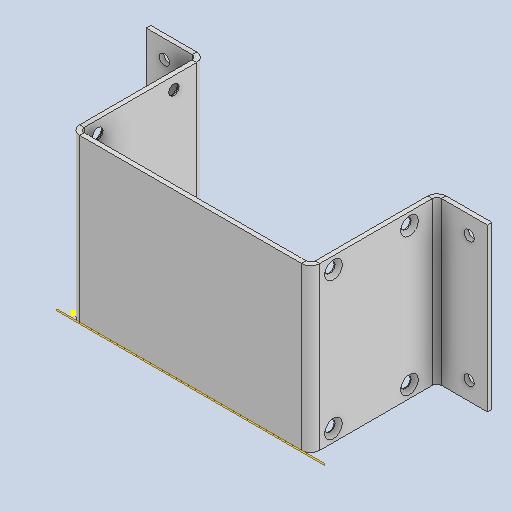
# Autodesk Inventor part: Top
Saved by Autodesk Inventor 2024 (Build 280153000, 153)
## iProperties
Created: 2025-10-29
Part Number: Top
Material: 일반
Document SubType Name: Sheet Metal
Designer: alexi
Density: 1 g/cm^3
Appearance: 기본값
Sheet Metal Rule: 기본값
Author: alexi
Autodesk Inventor part; units mm, degrees
ref_plane "YZ Plane" through (0, 0, 0) normal (1, 0, 0) x (0, 1, 0)
ref_plane "XZ Plane" through (0, 0, 0) normal (0, 1, 0) x (-1, 0, 0)
ref_plane "XY Plane" through (0, 0, 0) normal (0, 0, 1) x (1, 0, 0)
ref_plane "작업 평면1" through (0, 0, 0) normal (0, 0, 1) x (1, 0, 0)
sketch "스케치1" plane through (0, 0, 0) normal (0, 0, 1) x (1, 0, 0)
  line L0 (80, 11.5982) -> (80.0982, 11.5982) projected
  line L1 (80.0982, 41.5982) -> (80, 41.5982) projected
  line L2 (0, 41.5982) -> (-0.0982, 41.5982) projected
  line L3 (5, -0.0088) -> (3.5, -0.0088)
  line L4 (3.5, -0.0088) -> (3.5, 53.2053)
  line L5 (3.5, 53.2053) -> (5, 53.2053)
  line L6 (5, 53.2053) -> (5, -0.0088)
  line L7 (3.5, -0.0088) -> (0, -0.0088)
  line L8 (0, -0.0088) -> (0, 53.2053)
  line L9 (0, 53.2053) -> (3.5, 53.2053)
  line L10 (3.5, 53.2053) -> (3.5, -0.0088)
  line L11 (0, -0.0088) -> (-36.9, -0.0088)
  line L12 (-36.9, -0.0088) -> (-36.9, 53.2053)
  line L13 (-36.9, 53.2053) -> (0, 53.2053)
  line L14 (0, 53.2053) -> (0, -0.0088)
  line L15 (5, 53.2053) -> (5, -0.0088)
  line L16 (75, -0.0088) -> (76.5, -0.0088)
  line L17 (76.5, -0.0088) -> (76.5, 53.2053)
  line L18 (76.5, 53.2053) -> (75, 53.2053)
  line L19 (75, 53.2053) -> (75, -0.0088)
  line L20 (76.5, -0.0088) -> (80, -0.0088)
  line L21 (80, -0.0088) -> (80, 53.2053)
  line L22 (80, 53.2053) -> (76.5, 53.2053)
  line L23 (76.5, 53.2053) -> (76.5, -0.0088)
  line L24 (80, -0.0088) -> (116.9, -0.0088)
  line L25 (116.9, -0.0088) -> (116.9, 53.2053)
  line L26 (116.9, 53.2053) -> (80, 53.2053)
  line L27 (80, 53.2053) -> (80, -0.0088)
  line L28 (5, -0.0088) -> (75, -0.0088) projected
  line L29 (75, 53.2053) -> (5, 53.2053) projected
  line L30 (-36.9, -0.0088) -> (-40.4, -0.0088)
  line L31 (-40.4, -0.0088) -> (-40.4, 53.2053)
  line L32 (-40.4, 53.2053) -> (-36.9, 53.2053)
  line L33 (-36.9, 53.2053) -> (-36.9, -0.0088)
  line L34 (-40.4, -0.0088) -> (-55.4, -0.0088)
  line L35 (-55.4, -0.0088) -> (-55.4, 53.2053)
  line L36 (-55.4, 53.2053) -> (-40.4, 53.2053)
  line L37 (-40.4, 53.2053) -> (-40.4, -0.0088)
  line L38 (116.9, -0.0088) -> (120.4, -0.0088)
  line L39 (120.4, -0.0088) -> (120.4, 53.2053)
  line L40 (120.4, 53.2053) -> (116.9, 53.2053)
  line L41 (116.9, 53.2053) -> (116.9, -0.0088)
  line L42 (120.4, -0.0088) -> (135.4, -0.0088)
  line L43 (135.4, -0.0088) -> (135.4, 53.2053)
  line L44 (135.4, 53.2053) -> (120.4, 53.2053)
  line L45 (120.4, 53.2053) -> (120.4, -0.0088)
  point P0 (0, 0)
  dimension "d0" = 1.5
  dimension "d1" = 3.5
  dimension "d2" = 36.9
  dimension "d3" = 1.5
  dimension "d4" = 3.5
  dimension "d5" = 36.9
  dimension "d33" = 3.5
  dimension "d34" = 3.5
  dimension "d35" = 15
  dimension "d36" = 15
  constraints: 82 end point, 21 equal length, 10 horizontal, 10 perpendicular, 6 point on line
  measures "d0" distance of L5.end L4.end
  measures "d1" distance of L8.end L9.end
  measures "d2" distance of L12.end L13.end
  measures "d3" distance of L18.end L17.end
  measures "d4" distance of L21.end L22.end
  measures "d5" distance of L21.end L25.end
  measures "d33" distance of L12.end L31.end
  measures "d34" distance of L39.end L40.end
  measures "d35" distance of L35.end L36.end
  measures "d36" distance of L43.end L44.end
extrude "판1" add sketch "스케치1" against normal blind 1.5
sketch "스케치2" plane through (0, 0, -1.5) normal (0, 0, -1) x (-1, 0, 0)
  line L0 (-5, 53.2053) -> (-5, -0.0088) projected
  line L1 (-3.5, -0.0088) -> (-3.5, 53.2053) projected
  line L2 (-75, 53.2053) -> (-75, -0.0088) projected
  line L3 (-76.5, 53.2053) -> (-76.5, -0.0088) projected
  point P0 (0, 0)
  constraints: 1 other
fold "접기3" angle 90 bend radius 1.5 thickness 1.5 k factor 0.44 line from (-36.9, -0.0088, 0) to (-36.9, 53.2053, 0) line at bend start moving side (-1, 0, 0) folds toward (0, 0, 1)
fold "접기4" angle 90 bend radius 1.5 thickness 1.5 k factor 0.44 line from (116.9, -0.0088, 0) to (116.9, 53.2053, 0) line at bend start moving side (1, 0, 0) folds toward (0, 0, 1)
fold "접기5" angle 90 bend radius 1.5 thickness 1.5 k factor 0.44 line from (76.5, 53.2053, -1.5) to (76.5, -0.0088, -1.5) line at bend start moving side (1, 0, 0) folds toward (0, 0, -1)
fold "접기6" angle 90 bend radius 1.5 thickness 1.5 k factor 0.44 line from (3.5, -0.0088, -1.5) to (3.5, 53.2053, -1.5) line at bend start moving side (-1, 0, 0) folds toward (0, 0, -1)
sketch "스케치5" plane through (0.5, 53.2053, -40.0071) normal (-1, 0, 0) x (0, 0, 1)
  circle A0 centre (32.5071, -4) radius 1.2295 projected
  circle A1 centre (7.5071, -4) radius 1.2295 projected
  circle A2 centre (7.5071, -49.2142) radius 1.2295 projected
  circle A3 centre (32.5071, -49.2142) radius 1.2295 projected
  point P0 (40.0071, -53.2053)
  constraints: 4 coincident
hole "구멍3" at (0.5, 49.2053, -7.5) at (0.5, 49.2053, -32.5) at (0.5, 3.9912, -32.5) at (0.5, 3.9912, -7.5) direction (1, 0, 0) diameter 3.4 depth 1.5 tip angle 118 countersink diameter 5.8 countersink angle 90
sketch "스케치6" plane through (79.5, -0.0088, -3) normal (1, 0, 0) x (0, 0, -1)
  circle A0 centre (4.5, 4) radius 1.2295 projected
  circle A1 centre (29.5, 4) radius 1.2295 projected
  circle A2 centre (29.5, 49.2142) radius 1.2295 projected
  circle A3 centre (4.5, 49.2142) radius 1.2295 projected
  point P0 (-3, 0.0088)
  constraints: 4 coincident
hole "구멍4" at (79.5, 3.9912, -7.5) at (79.5, 3.9912, -32.5) at (79.5, 49.2053, -32.5) at (79.5, 49.2053, -7.5) at (79.5, 3.9912, -7.5) at (79.5, 3.9912, -32.5) at (79.5, 49.2053, -32.5) direction (-1, 0, 0) diameter 3.4 depth 1.5 tip angle 118 countersink diameter 5.8 countersink angle 90
sketch "스케치7" plane through (-16.1071, 53.2053, -41.5071) normal (0, 0, 1) x (1, 0, 0)
  line L0 (0, 0) -> (0, -53.2142) projected
  line L1 (15.1071, 0) -> (0, 0) projected
  line L2 (0, -53.2142) -> (15.1071, -53.2142) projected
  point P0 (16.1071, -53.2053)
  point P1 (6, -6)
  point P2 (6, -47.2142)
  dimension "d75" = 6
  dimension "d76" = 6
  dimension "d77" = 6
  dimension "d78" = 6
  measures "d75" distance from line of L0 point (6, -6)
  measures "d76" distance from line of L1 point (6, -6)
  measures "d77" distance from line of L2 point (6, -47.214)
  measures "d78" distance from line of L0 point (6, -47.214)
sketch "스케치8" plane through (81, -0.0088, -41.5071) normal (0, 0, 1) x (1, 0, 0)
  line L0 (15.1071, 0) -> (15.1071, 53.2142) projected
  line L1 (15.1071, 53.2142) -> (0, 53.2142) projected
  line L2 (0, 0) -> (15.1071, 0) projected
  point P0 (-81, 0.0088)
  point P1 (9.1071, 47.2142)
  point P2 (9.1071, 6)
  dimension "d79" = 6
  dimension "d80" = 6
  dimension "d81" = 6
  dimension "d82" = 6
  measures "d79" distance from line of L0 point (9.107, 47.214)
  measures "d80" distance from line of L1 point (9.107, 47.214)
  measures "d81" distance from line of L2 point (9.107, 6)
  measures "d82" distance from line of L0 point (9.107, 6)
hole "구멍5" at (-10.1071, 47.2053, -41.5071) at (-10.1071, 5.9912, -41.5071) direction (0, 0, -1) diameter 3.4 depth 1.5 tip angle 118
hole "구멍6" at (90.1071, 47.2053, -41.5071) at (90.1071, 5.9912, -41.5071) direction (0, 0, -1) diameter 3.4 depth 1.5 tip angle 118
equation "\"d0\" = d3"
equation "\"d1\" = d4"
equation "\"d2\" = d5"
equation "\"d33\" = d4"
equation "\"d34\" = d4"
equation "\"d37\" = BendReliefWidth"
equation "\"d38\" = BendReliefDepth"
equation "\"d39\" = MinimumRemnant"
equation "\"d40\" = TransitionRadius"
equation "\"d43\" = BendReliefWidth"
equation "\"d44\" = BendReliefDepth"
equation "\"d45\" = MinimumRemnant"
equation "\"d46\" = TransitionRadius"
equation "\"d49\" = BendReliefWidth"
equation "\"d50\" = BendReliefDepth"
equation "\"d51\" = MinimumRemnant"
equation "\"d52\" = TransitionRadius"
equation "\"d55\" = BendReliefWidth"
equation "\"d56\" = BendReliefDepth"
equation "\"d57\" = MinimumRemnant"
equation "\"d58\" = TransitionRadius"
equation "\"TransitionRadius\" = BendRadius"
equation "\"BendReliefWidth\" = 1.5"
equation "\"BendReliefDepth\" = 0.75"
equation "\"MinimumRemnant\" = 3"
equation "\"BendRadius\" = 1.5"
